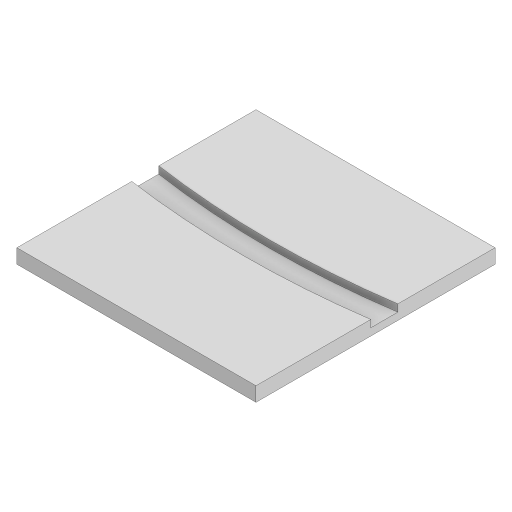
# Autodesk Inventor part: big_curve
Saved by Autodesk Inventor 2023 (Build 270158000, 158)
## iProperties
Created: 2022-07-12
Part Number: big_curve
Material: Generic
Document SubType Name: Modeling
Designer: Derm
Density: 1 g/cm^3
Appearance: Default
Author: Derm
Autodesk Inventor part; units mm, degrees
ref_plane "YZ Plane" through (0, 0, 0) normal (1, 0, 0) x (0, 1, 0)
ref_plane "XZ Plane" through (0, 0, 0) normal (0, 1, 0) x (-1, 0, 0)
ref_plane "XY Plane" through (0, 0, 0) normal (0, 0, 1) x (1, 0, 0)
sketch "Sketch1" plane through (0, 0, 0) normal (0, 1, 0) x (-1, 0, 0)
  line L0 (-50000, 50000) -> (50000, 50000)
  line L1 (50000, 50000) -> (50000, -50000)
  line L2 (50000, -50000) -> (-50000, -50000)
  line L3 (-50000, -50000) -> (-50000, 50000)
  line L4 (-50000, 50000) -> (50000, -50000) construction
  line L5 (50000, 50000) -> (-50000, -50000) construction
  point P0 (0, 0)
  dimension "d0" = 100000
  dimension "d1" = 100000
  constraints: 12 end point, 2 midpoint, 2 parallel, 1 horizontal, 1 perpendicular
  measures "d0" distance of L0.end L1.end
  measures "d1" distance of L1.end L2.end
extrude "Extrusion1" add sketch "Sketch1" against normal blind 3000
sketch "Sketch2" plane through (0, 0, 0) normal (0, 1, 0) x (1, 0, 0)
  line L0 (-50000, 50000) -> (50000, 50000) projected
  line L1 (50000, 50000) -> (50000, -50000) projected
  arc A0 (-50000, 9325.0108) -> (50000, 9325.0108) centre (0, 347830.301) ccw
  line L2 (50000, 50000) -> (-50000, 50000) projected
  line L3 (-50000, 50000) -> (-50000, -50000) projected
  line L4 (-50000, -50000) -> (50000, -50000) projected
  line L5 (50000, -50000) -> (50000, 50000) projected
  arc A1 (-50000, -1974.3373) -> (50000, -1974.3373) centre (0, 347830.301) ccw
  point P0 (0, 0)
  point P1 (50000, -1974.3373)
  constraints: 5 point on line, 4 point on circle, 2 centre point
extrude "Extrusion2" add sketch "Sketch2" along normal blind 3000 contours L0 L1 A0 L3 | A1 L1 L4 L3
body "Solid1"
